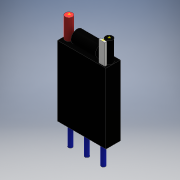
# Autodesk Inventor part: ESC
Saved by Autodesk Inventor 2016 (Build 200138000, 138)
## iProperties
Created: 2015-09-20
Part Number: ESC
Material: Generic
Document SubType Name: Modeling
Designer: Artur
Density: 1 g/cm^3
Appearance: Default
Mass: 6.48699 g
Surface Area: 37.275 cm^2
Volume: 6.48699 cm^3
Author: Artur
Autodesk Inventor part; units mm, degrees
ref_plane "YZ Plane" through (0, 0, 0) normal (1, 0, 0) x (0, 1, 0)
sketch "Sketch1" plane through (0, 0, 0) normal (0, 1, 0) x (-1, 0, 0)
  line L0 (23.5, 0) -> (0, 0)
  line L1 (0, 0) -> (0, -34)
  line L2 (0, -34) -> (23.5, -34)
  line L3 (23.5, -34) -> (23.5, 0)
  dimension "d0" = 34
  dimension "d1" = 23.5
  constraints: 8 end point, 2 parallel, 1 coincident, 1 horizontal, 1 perpendicular
  measures "d0" distance of L0.end L1.end
  measures "d1" distance of L1.end L2.end
extrude "Extrusion1" add sketch "Sketch1" along normal blind 7
ref_plane "Work Plane1" through (-17.5, 0, -34) normal (-1, 0, 0) x (0, 0, 1)
sketch "Sketch2" plane through (-17.5, 0, -34) normal (-1, 0, 0) x (0, 0, 1)
  circle A0 centre (37.1, 3.4714) radius 3
  line L0 (34, 0) -> (34, 7) projected
  dimension "d5" = 6
  dimension "d6" = 3.1
  constraints: 1 centre point
  measures "d5" diameter of A0
  measures "d6" distance from line of L0 A0.centre
extrude "Extrusion2" add sketch "Sketch2" against normal blind 12 separate body
sketch "Sketch3" plane through (0, 7, 0) normal (0, 1, 0) x (1, 0, 0)
  line L0 (-23.5, 0) -> (0, 0) construction
  line L1 (0, 34) -> (-23.5, 34) construction
  line L2 (-22, 0) -> (-22, 34)
  line L3 (-22, 34) -> (-21, 34)
  line L4 (-21, 34) -> (-21, 0)
  line L5 (-21, 0) -> (-22, 0)
  line L6 (-23.5, 34) -> (-23.5, 0) projected
  line L7 (-18.75, 0) -> (-19.75, 0)
  line L8 (-18.75, 34) -> (-18.75, 0)
  line L9 (-19.75, 0) -> (-19.75, 34)
  line L10 (-19.75, 34) -> (-18.75, 34)
  line L11 (-16.5, 0) -> (-17.5, 0)
  line L12 (-16.5, 34) -> (-16.5, 0)
  line L13 (-17.5, 0) -> (-17.5, 34)
  line L14 (-17.5, 34) -> (-16.5, 34)
  line L15 (-14.25, 0) -> (-15.25, 0)
  line L16 (-14.25, 34) -> (-14.25, 0)
  line L17 (-15.25, 0) -> (-15.25, 34)
  line L18 (-15.25, 34) -> (-14.25, 34)
  line L19 (-12, 0) -> (-13, 0)
  line L20 (-12, 34) -> (-12, 0)
  line L21 (-13, 0) -> (-13, 34)
  line L22 (-13, 34) -> (-12, 34)
  line L23 (-9.75, 0) -> (-10.75, 0)
  line L24 (-9.75, 34) -> (-9.75, 0)
  line L25 (-10.75, 0) -> (-10.75, 34)
  line L26 (-10.75, 34) -> (-9.75, 34)
  line L27 (-7.5, 0) -> (-8.5, 0)
  line L28 (-7.5, 34) -> (-7.5, 0)
  line L29 (-8.5, 0) -> (-8.5, 34)
  line L30 (-8.5, 34) -> (-7.5, 34)
  dimension "d9" = 1
  dimension "d10" = 1.5
  dimension "d13" = 2.25
  constraints: 56 end point, 3 perpendicular, 2 point on line, 1 horizontal, 1 vertical, 48 other
  measures "d9" distance of L2.end L3.end
  measures "d10" distance from line of L6 L2.start
  measures "d13" distance of L2.start L7.end
extrude "Extrusion3" add sketch "Sketch3" along normal blind 1 bodies 1
ref_plane "Work Plane2" through (-21, 8, 0) normal (0, 1, 0) x (1, 0, 0)
sketch "Sketch4" plane through (-21, 8, 0) normal (0, 1, 0) x (1, 0, 0)
  line L0 (15.8525, 1.5) -> (15.8525, 17.0203) construction
  line L1 (15.8525, 17.0203) -> (19.5, 17.0203) construction
  line L2 (19.5, 17.0203) -> (19.5, 1.5) construction
  line L3 (19.5, 1.5) -> (15.8525, 1.5) construction
  line L4 (21, 0) -> (21, 34) projected
  line L5 (13.5, 0) -> (21, 0) projected
  line L6 (2.3, 7) -> (2.3, 27.0073) construction
  line L7 (2.3, 27.0073) -> (4.301, 27.0073) construction
  line L8 (4.301, 27.0073) -> (4.301, 7) construction
  line L9 (4.301, 7) -> (2.3, 7) construction
  line L10 (2.25, 0) -> (3.5, 0) projected
  line L11 (-2.5, 34) -> (-2.5, 0) projected
  line L12 (5.6079, 8.0877) -> (2.7425, 8.0877)
  line L13 (2.7425, 8.0877) -> (2.7425, 6.9974)
  line L14 (2.7425, 6.9974) -> (2.3579, 6.9974)
  line L15 (2.3579, 6.9974) -> (2.3579, 9.61)
  line L16 (2.3579, 9.61) -> (2.7425, 9.61)
  line L17 (2.7425, 9.61) -> (2.7425, 8.5197)
  line L18 (2.7425, 8.5197) -> (5.6079, 8.5197)
  line L19 (5.6079, 8.5197) -> (5.6079, 8.0877)
  spline S0 degree 2 poles (5.6764, 11.0744) (5.6764, 10.7873) (5.5263, 10.3606) (5.3762, 10.2105) knots 0 0 0 1 2 2 2
  spline S1 degree 2 poles (5.3762, 10.2105) (5.2076, 10.0393) (4.7335, 9.8997) (4.3859, 9.8997) knots 0 0 0 1 2 2 2
  line L20 (4.3859, 9.8997) -> (2.3579, 9.8997)
  line L21 (2.3579, 9.8997) -> (2.3579, 10.3316)
  line L22 (2.3579, 10.3316) -> (4.3859, 10.3316)
  spline S2 degree 2 poles (4.3859, 10.3316) (4.6124, 10.3316) (4.9179, 10.3896) (5.0417, 10.4712) knots 0 0 0 1 2 2 2
  spline S3 degree 2 poles (5.0417, 10.4712) (5.1734, 10.5581) (5.3077, 10.8584) (5.3077, 11.0744) knots 0 0 0 1 2 2 2
  spline S4 degree 2 poles (5.3077, 11.0744) (5.3077, 11.2771) (5.1734, 11.5932) (5.0417, 11.6801) knots 0 0 0 1 2 2 2
  spline S5 degree 2 poles (5.0417, 11.6801) (4.9179, 11.7618) (4.615, 11.8197) (4.3964, 11.8197) knots 0 0 0 1 2 2 2
  line L23 (4.3964, 11.8197) -> (2.3579, 11.8197)
  line L24 (2.3579, 11.8197) -> (2.3579, 12.2516)
  line L25 (2.3579, 12.2516) -> (4.3859, 12.2516)
  spline S6 degree 2 poles (4.3859, 12.2516) (4.7256, 12.2516) (5.2103, 12.1147) (5.3762, 11.9408) knots 0 0 0 1 2 2 2
  spline S7 degree 2 poles (5.3762, 11.9408) (5.5289, 11.7855) (5.6764, 11.3746) (5.6764, 11.0744) knots 0 0 0 1 2 2 2
  line L26 (5.6079, 15.3857) -> (5.6079, 14.8248)
  line L27 (5.6079, 14.8248) -> (4.3148, 13.7976)
  line L28 (4.3148, 13.7976) -> (4.3148, 13.3025)
  line L29 (4.3148, 13.3025) -> (5.6079, 13.3025)
  line L30 (5.6079, 13.3025) -> (5.6079, 12.8705)
  line L31 (5.6079, 12.8705) -> (2.3579, 12.8705)
  line L32 (2.3579, 12.8705) -> (2.3579, 13.7081)
  spline S8 degree 2 poles (2.3579, 13.7081) (2.3579, 13.9872) (2.4185, 14.3639) (2.5291, 14.535) knots 0 0 0 1 2 2 2
  spline S9 degree 2 poles (2.5291, 14.535) (2.6397, 14.7062) (2.9848, 14.9038) (3.2402, 14.9038) knots 0 0 0 1 2 2 2
  spline S10 degree 2 poles (3.2402, 14.9038) (3.5958, 14.9038) (4.0778, 14.5403) (4.1936, 14.2295) knots 0 0 0 1 2 2 2
  line L33 (4.1936, 14.2295) -> (5.6079, 15.3857)
  spline S11 degree 2 poles (3.2745, 14.4534) (3.1323, 14.4534) (2.9137, 14.3533) (2.8425, 14.248) knots 0 0 0 1 2 2 2
  spline S12 degree 2 poles (2.8425, 14.248) (2.782, 14.1558) (2.7319, 13.9109) (2.7319, 13.7318) knots 0 0 0 1 2 2 2
  line L34 (2.7319, 13.7318) -> (2.7319, 13.3025)
  line L35 (2.7319, 13.3025) -> (3.954, 13.3025)
  line L36 (3.954, 13.3025) -> (3.954, 13.6817)
  spline S13 degree 2 poles (3.954, 13.6817) (3.954, 13.8687) (3.8881, 14.1663) (3.7854, 14.269) knots 0 0 0 1 2 2 2
  spline S14 degree 2 poles (3.7854, 14.269) (3.6959, 14.3639) (3.443, 14.4534) (3.2745, 14.4534) knots 0 0 0 1 2 2 2
  line L37 (5.6079, 17.9694) -> (5.6079, 17.4848)
  line L38 (5.6079, 17.4848) -> (2.8057, 16.0468)
  line L39 (2.8057, 16.0468) -> (5.6079, 16.0468)
  line L40 (5.6079, 16.0468) -> (5.6079, 15.6438)
  line L41 (5.6079, 15.6438) -> (2.3579, 15.6438)
  line L42 (2.3579, 15.6438) -> (2.3579, 16.2575)
  line L43 (2.3579, 16.2575) -> (4.9311, 17.5665)
  line L44 (4.9311, 17.5665) -> (2.3579, 17.5665)
  line L45 (2.3579, 17.5665) -> (2.3579, 17.9694)
  line L46 (2.3579, 17.9694) -> (5.6079, 17.9694)
  line L47 (5.6079, 19.7603) -> (5.6079, 18.5014)
  line L48 (5.6079, 18.5014) -> (5.2761, 18.5014)
  line L49 (5.2761, 18.5014) -> (5.2761, 18.9149)
  line L50 (5.2761, 18.9149) -> (2.6898, 18.9149)
  line L51 (2.6898, 18.9149) -> (2.6898, 18.5014)
  line L52 (2.6898, 18.5014) -> (2.3579, 18.5014)
  line L53 (2.3579, 18.5014) -> (2.3579, 19.7603)
  line L54 (2.3579, 19.7603) -> (2.6898, 19.7603)
  line L55 (2.6898, 19.7603) -> (2.6898, 19.3468)
  line L56 (2.6898, 19.3468) -> (5.2761, 19.3468)
  line L57 (5.2761, 19.3468) -> (5.2761, 19.7603)
  line L58 (5.2761, 19.7603) -> (5.6079, 19.7603)
  spline S15 degree 2 poles (5.6712, 21.6566) (5.6712, 21.3116) (5.4605, 20.7401) (5.2471, 20.5346) knots 0 0 0 1 2 2 2
  spline S16 degree 2 poles (5.2471, 20.5346) (5.0312, 20.3292) (4.3938, 20.1106) (3.9803, 20.1106) knots 0 0 0 1 2 2 2
  spline S17 degree 2 poles (3.9803, 20.1106) (3.5879, 20.1106) (2.9663, 20.3318) (2.7451, 20.5373) knots 0 0 0 1 2 2 2
  spline S18 degree 2 poles (2.7451, 20.5373) (2.5318, 20.7348) (2.3, 21.3142) (2.3, 21.6592) knots 0 0 0 1 2 2 2
  spline S19 degree 2 poles (2.3, 21.6592) (2.3, 21.8252) (2.3474, 22.1254) (2.3895, 22.2624) knots 0 0 0 1 2 2 2
  spline S20 degree 2 poles (2.3895, 22.2624) (2.4212, 22.373) (2.537, 22.6416) (2.5792, 22.7233) knots 0 0 0 1 2 2 2
  line L59 (2.5792, 22.7233) -> (3.1006, 22.7233)
  line L60 (3.1006, 22.7233) -> (3.1006, 22.6864)
  spline S21 degree 2 poles (3.1006, 22.6864) (3.0295, 22.6047) (2.9005, 22.4335) (2.8267, 22.2755) knots 0 0 0 1 2 2 2
  spline S22 degree 2 poles (2.8267, 22.2755) (2.7609, 22.1438) (2.674, 21.8041) (2.674, 21.6092) knots 0 0 0 1 2 2 2
  spline S23 degree 2 poles (2.674, 21.6092) (2.674, 21.1404) (3.3798, 20.561) (3.9671, 20.561) knots 0 0 0 1 2 2 2
  spline S24 degree 2 poles (3.9671, 20.561) (4.2937, 20.561) (4.7836, 20.7137) (4.9521, 20.8586) knots 0 0 0 1 2 2 2
  spline S25 degree 2 poles (4.9521, 20.8586) (5.1207, 20.9982) (5.2972, 21.3932) (5.2972, 21.6408) knots 0 0 0 1 2 2 2
  spline S26 degree 2 poles (5.2972, 21.6408) (5.2972, 21.8225) (5.2445, 22.186) (5.1918, 22.3098) knots 0 0 0 1 2 2 2
  line L61 (5.1918, 22.3098) -> (4.3517, 22.3098)
  line L62 (4.3517, 22.3098) -> (4.3517, 21.5565)
  line L63 (4.3517, 21.5565) -> (3.9724, 21.5565)
  line L64 (3.9724, 21.5565) -> (3.9724, 22.7364)
  line L65 (3.9724, 22.7364) -> (5.392, 22.7364)
  spline S27 degree 2 poles (5.392, 22.7364) (5.4288, 22.6548) (5.5421, 22.3756) (5.5763, 22.2571) knots 0 0 0 1 2 2 2
  spline S28 degree 2 poles (5.5763, 22.2571) (5.6237, 22.0964) (5.6712, 21.8383) (5.6712, 21.6566) knots 0 0 0 1 2 2 2
  line L66 (2.3579, 25.5545) -> (4.1699, 24.4562)
  line L67 (4.1699, 24.4562) -> (5.6079, 24.4562)
  line L68 (5.6079, 24.4562) -> (5.6079, 24.0243)
  line L69 (5.6079, 24.0243) -> (4.2147, 24.0243)
  line L70 (4.2147, 24.0243) -> (2.3579, 22.9261)
  line L71 (2.3579, 22.9261) -> (2.3579, 23.4054)
  line L72 (2.3579, 23.4054) -> (3.788, 24.2429)
  line L73 (3.788, 24.2429) -> (2.3579, 25.0962)
  line L74 (2.3579, 25.0962) -> (2.3579, 25.5545)
  line L75 (19.4263, 1.4773) -> (15.9263, 2.6572)
  line L76 (15.9263, 2.6572) -> (15.9263, 3.2301)
  line L77 (15.9263, 3.2301) -> (19.4263, 4.41)
  line L78 (19.4263, 4.41) -> (19.4263, 3.9194)
  line L79 (19.4263, 3.9194) -> (18.4477, 3.6017)
  line L80 (18.4477, 3.6017) -> (18.4477, 2.2658)
  line L81 (18.4477, 2.2658) -> (19.4263, 1.9481)
  line L82 (19.4263, 1.9481) -> (19.4263, 1.4773)
  line L83 (18.0506, 3.4741) -> (16.4028, 2.9323)
  line L84 (16.4028, 2.9323) -> (18.0506, 2.3934)
  line L85 (18.0506, 2.3934) -> (18.0506, 3.4741)
  line L86 (19.4263, 4.7419) -> (15.9263, 4.7419)
  line L87 (15.9263, 4.7419) -> (15.9263, 6.9315)
  line L88 (15.9263, 6.9315) -> (16.3404, 6.9315)
  line L89 (16.3404, 6.9315) -> (16.3404, 5.2071)
  line L90 (16.3404, 5.2071) -> (17.299, 5.2071)
  line L91 (17.299, 5.2071) -> (17.299, 6.8152)
  line L92 (17.299, 6.8152) -> (17.7131, 6.8152)
  line L93 (17.7131, 6.8152) -> (17.7131, 5.2071)
  line L94 (17.7131, 5.2071) -> (19.0122, 5.2071)
  line L95 (19.0122, 5.2071) -> (19.0122, 6.9315)
  line L96 (19.0122, 6.9315) -> (19.4263, 6.9315)
  line L97 (19.4263, 6.9315) -> (19.4263, 4.7419)
  line L98 (18.1074, 8.6248) -> (18.1074, 7.3002)
  line L99 (18.1074, 7.3002) -> (17.6819, 7.3002)
  line L100 (17.6819, 7.3002) -> (17.6819, 8.6248)
  line L101 (17.6819, 8.6248) -> (18.1074, 8.6248)
  line L102 (19.4263, 11.2484) -> (19.4263, 9.09)
  line L103 (19.4263, 9.09) -> (18.9299, 9.09)
  spline S29 degree 2 poles (18.9299, 9.09) (18.7115, 9.3225) (18.3059, 9.7366) (18.0875, 9.9352) knots 0 0 0 1 2 2 2
  spline S30 degree 2 poles (18.0875, 9.9352) (17.6479, 10.3351) (17.1203, 10.6272) (16.8395, 10.6272) knots 0 0 0 1 2 2 2
  spline S31 degree 2 poles (16.8395, 10.6272) (16.6921, 10.6272) (16.4708, 10.5365) (16.3999, 10.4542) knots 0 0 0 1 2 2 2
  spline S32 degree 2 poles (16.3999, 10.4542) (16.329, 10.372) (16.2581, 10.1564) (16.2581, 10.0259) knots 0 0 0 1 2 2 2
  spline S33 degree 2 poles (16.2581, 10.0259) (16.2581, 9.9011) (16.3205, 9.6459) (16.3687, 9.5296) knots 0 0 0 1 2 2 2
  spline S34 degree 2 poles (16.3687, 9.5296) (16.4084, 9.4303) (16.5219, 9.2459) (16.5616, 9.1892) knots 0 0 0 1 2 2 2
  line L104 (16.5616, 9.1892) -> (16.5616, 9.1637)
  line L105 (16.5616, 9.1637) -> (16.0624, 9.1637)
  spline S35 degree 2 poles (16.0624, 9.1637) (15.9915, 9.3083) (15.8525, 9.8274) (15.8525, 10.06) knots 0 0 0 1 2 2 2
  spline S36 degree 2 poles (15.8525, 10.06) (15.8525, 10.5506) (16.3716, 11.1037) (16.814, 11.1037) knots 0 0 0 1 2 2 2
  spline S37 degree 2 poles (16.814, 11.1037) (17.0211, 11.1037) (17.3671, 11.0073) (17.5146, 10.9222) knots 0 0 0 1 2 2 2
  spline S38 degree 2 poles (17.5146, 10.9222) (17.6677, 10.8371) (17.9684, 10.5904) (18.113, 10.4542) knots 0 0 0 1 2 2 2
  spline S39 degree 2 poles (18.113, 10.4542) (18.3541, 10.233) (18.8703, 9.6912) (19.0207, 9.5296) knots 0 0 0 1 2 2 2
  line L106 (19.0207, 9.5296) -> (19.0207, 11.2484)
  line L107 (19.0207, 11.2484) -> (19.4263, 11.2484)
  spline S40 degree 2 poles (18.3144, 13.8379) (18.5669, 13.8379) (18.998, 13.6763) (19.1568, 13.5288) knots 0 0 0 1 2 2 2
  spline S41 degree 2 poles (19.1568, 13.5288) (19.3156, 13.3813) (19.5, 12.9417) (19.5, 12.6694) knots 0 0 0 1 2 2 2
  spline S42 degree 2 poles (19.5, 12.6694) (19.5, 12.4198) (19.3894, 11.9319) (19.3015, 11.7532) knots 0 0 0 1 2 2 2
  line L108 (19.3015, 11.7532) -> (18.8051, 11.7532)
  line L109 (18.8051, 11.7532) -> (18.8051, 11.7873)
  spline S43 degree 2 poles (18.8051, 11.7873) (18.8448, 11.8412) (18.9469, 12.0425) (18.9923, 12.1645) knots 0 0 0 1 2 2 2
  spline S44 degree 2 poles (18.9923, 12.1645) (19.0405, 12.3035) (19.0944, 12.5332) (19.0944, 12.6779) knots 0 0 0 1 2 2 2
  spline S45 degree 2 poles (19.0944, 12.6779) (19.0944, 12.8197) (18.9923, 13.0863) (18.8817, 13.1827) knots 0 0 0 1 2 2 2
  spline S46 degree 2 poles (18.8817, 13.1827) (18.7767, 13.2707) (18.4988, 13.3614) (18.3116, 13.3614) knots 0 0 0 1 2 2 2
  spline S47 degree 2 poles (18.3116, 13.3614) (18.1244, 13.3614) (17.8861, 13.2593) (17.8067, 13.1629) knots 0 0 0 1 2 2 2
  spline S48 degree 2 poles (17.8067, 13.1629) (17.7188, 13.0636) (17.6451, 12.7686) (17.6451, 12.59) knots 0 0 0 1 2 2 2
  spline S49 degree 2 poles (17.6451, 12.59) (17.6451, 12.3971) (17.7046, 12.0142) (17.7301, 11.8979) knots 0 0 0 1 2 2 2
  line L110 (17.7301, 11.8979) -> (15.9263, 11.8979)
  line L111 (15.9263, 11.8979) -> (15.9263, 13.8181)
  line L112 (15.9263, 13.8181) -> (16.3375, 13.8181)
  line L113 (16.3375, 13.8181) -> (16.3375, 12.3489)
  line L114 (16.3375, 12.3489) -> (17.2707, 12.3489)
  spline S50 degree 2 poles (17.2707, 12.3489) (17.2593, 12.434) (17.2508, 12.5985) (17.2508, 12.6665) knots 0 0 0 1 2 2 2
  spline S51 degree 2 poles (17.2508, 12.6665) (17.2508, 12.936) (17.3387, 13.3075) (17.4692, 13.4777) knots 0 0 0 1 2 2 2
  spline S52 degree 2 poles (17.4692, 13.4777) (17.5997, 13.6507) (17.9968, 13.8379) (18.3144, 13.8379) knots 0 0 0 1 2 2 2
  line L115 (19.4263, 14.0648) -> (15.9263, 15.2447)
  line L116 (15.9263, 15.2447) -> (15.9263, 15.8177)
  line L117 (15.9263, 15.8177) -> (19.4263, 16.9976)
  line L118 (19.4263, 16.9976) -> (19.4263, 16.5069)
  line L119 (19.4263, 16.5069) -> (18.4477, 16.1892)
  line L120 (18.4477, 16.1892) -> (18.4477, 14.8533)
  line L121 (18.4477, 14.8533) -> (19.4263, 14.5357)
  line L122 (19.4263, 14.5357) -> (19.4263, 14.0648)
  line L123 (18.0506, 16.0616) -> (16.4028, 15.5199)
  line L124 (16.4028, 15.5199) -> (18.0506, 14.981)
  line L125 (18.0506, 14.981) -> (18.0506, 16.0616)
  dimension "d0" = 34
  dimension "d1" = 23.5
  dimension "d20" = 1.5
  dimension "d21" = 1.5
  dimension "d22" = 7
  dimension "d23" = 4.8
  constraints: 4 other
  measures "d20" distance between parallel lines of L4 L2
  measures "d21" distance between parallel lines of L5 L3
  measures "d22" distance between parallel lines of L10 L9
  measures "d23" distance between parallel lines of L11 L6
emboss "Emboss1" sketch "Sketch4" operation add depth 0.0001 direction (0, -1, 0)
sketch "Sketch5" plane through (0, 0, -34) normal (0, 0, -1) x (-1, 0, 0)
  line L0 (23.5, 0) -> (23.5, 7) construction
  line L1 (0, 0) -> (23.5, 0) construction
  circle A0 centre (19.75, 2.5) radius 1
  circle A1 centre (11.75, 2.5) radius 1
  circle A2 centre (3.75, 2.5) radius 1
  dimension "d26" = 2
  dimension "d27" = 2.5
  dimension "d28" = 3.75
  dimension "d31" = 8
  constraints: 3 centre point, 1 horizontal, 4 other
  measures "d26" diameter of A0
  measures "d27" distance from line of L1 A0.centre
  measures "d28" distance from line of L0 A0.centre
  measures "d31" distance of A0.centre A1.centre
extrude "Extrusion4" add sketch "Sketch5" along normal blind 10 separate body
sketch "Sketch6" plane through (-23.5, 0, 0) normal (0, 0, 1) x (1, 0, 0)
  circle A0 centre (2, 3.5) radius 1.75
  circle A1 centre (21.5, 3.5) radius 1.75
  line L0 (19.5, 1.5) -> (22.5, 1.5)
  line L1 (22.5, 1.5) -> (22.5, 0.5)
  line L2 (22.5, 0.5) -> (19.5, 0.5)
  line L3 (19.5, 0.5) -> (19.5, 1.5)
  line L4 (0, 0) -> (0, 7) projected
  line L5 (0, 0) -> (23.5, 0) projected
  line L6 (23.5, 0) -> (23.5, 7) projected
  dimension "d38" = 3.5
  dimension "d39" = 3.5
  dimension "d40" = 3
  dimension "d41" = 1
  dimension "d42" = 2
  dimension "d43" = 3.5
  dimension "d44" = 0.5
  dimension "d45" = 1
  dimension "d46" = 2
  dimension "d47" = 3.5
  constraints: 8 end point, 2 centre point, 2 parallel, 1 horizontal, 1 perpendicular
  measures "d38" diameter of A0
  measures "d39" diameter of A1
  measures "d40" distance of L1.end L2.end
  measures "d41" distance of L0.end L1.end
  measures "d42" distance from line of L4 A0.centre
  measures "d43" distance from line of L5 A0.centre
  measures "d44" distance between parallel lines of L5 L2
  measures "d45" distance between parallel lines of L6 L1
  measures "d46" distance from line of L6 A1.centre
  measures "d47" distance from line of L5 A1.centre
extrude "Extrusion5" add sketch "Sketch6" along normal blind 10 separate body contours A0 | A1
extrude "Extrusion6" add sketch "Sketch6" along normal blind 10 separate body contours L0 L1 L2 L3
sketch "Sketch7" plane through (-3.75, 2.5, -44) normal (0, 0, -1) x (-1, 0, 0)
  circle A0 centre (0, 0) radius 1 construction
  circle A1 centre (8, 0) radius 1 construction
  circle A2 centre (16, 0) radius 1 construction
  point P0 (-3.75, -2.5)
  constraints: 3 coincident
sketch "Sketch8" plane through (-2, 3.5, 10) normal (0, 0, 1) x (1, 0, 0)
  circle A0 centre (0, 0) radius 1.75 projected
  circle A1 centre (-19.5, 0) radius 1.75 projected
  point P0 (2, -3.5)
  constraints: 2 coincident
sketch "Sketch9" plane through (-23.5, 0, 10) normal (0, 0, 1) x (1, 0, 0)
  line L0 (19.5, 0.5) -> (22.5, 0.5) projected
  line L1 (22.5, 1.5) -> (19.5, 1.5) projected
  line L2 (19.5, 1.5) -> (19.5, 0.5) projected
  line L3 (22.5, 0.5) -> (22.5, 1.5) projected
  point P0 (23.5, 0)
  point P1 (21, 1)
  dimension "d52" = 1
  dimension "d53" = 3
  dimension "d54" = 0.5
  dimension "d55" = 1.5
  measures "d52" distance between parallel lines of L0 L1
  measures "d53" distance between parallel lines of L2 L3
  measures "d54" distance from line of L0 point (21, 1)
  measures "d55" distance from line of L3 point (21, 1)
equation "\"d54\" = 0.5 * d52"
equation "\"d55\" = 0.5 * d53"
